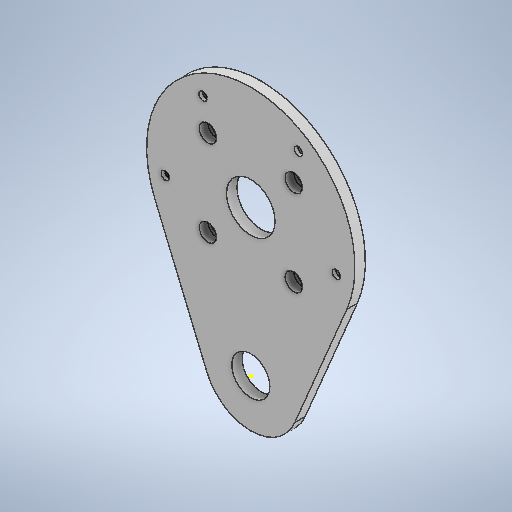
# Autodesk Inventor part: RT_ARM_MC_008_Capstand_Base
Saved by Autodesk Inventor 2025.3 (Build 293356000, 356)
## iProperties
Created: 2026-07-28
Part Number: RT_ARM_MC_008_Capstand_Base
Material: Generic
Document SubType Name: Modeling
Designer: louis
Density: 1 g/cm^3
Appearance: Default
Author: louis
Autodesk Inventor part; units mm, degrees
ref_plane "YZ Plane" through (0, 0, 0) normal (1, 0, 0) x (0, 1, 0)
ref_plane "XZ Plane" through (0, 0, 0) normal (0, 1, 0) x (-1, 0, 0)
ref_plane "XY Plane" through (0, 0, 0) normal (0, 0, 1) x (1, 0, 0)
sketch "Sketch1" plane through (0, 0, 0) normal (0, 0, 1) x (1, 0, 0)
  circle A0 centre (0, 0) radius 11
  circle A1 centre (0, 84) radius 14
  circle A2 centre (0, 0) radius 72 construction
  circle A3 centre (0, 84) radius 12 construction
  line L0 (0, 84) -> (0, 0) construction
  line L1 (-67.6579, 24.6255) -> (0, 0) construction
  line L2 (67.6579, 24.6255) -> (0, 0) construction
  circle A4 centre (0, 84) radius 35 construction
  line L3 (-60, 71.9226) -> (-60, 144)
  line L4 (-60, 144) -> (60, 144)
  line L5 (60, 144) -> (60, 71.9226)
  circle A5 centre (0, 0) radius 27.5
  line L6 (25.3583, -10.6399) -> (60, 71.9226)
  line L7 (-60, 71.9226) -> (-25.3583, -10.6399)
  line L8 (0, 0) -> (135.9462, -63.3927) construction
  line L9 (-24.7487, 59.2513) -> (24.7487, 59.2513) construction
  circle A6 centre (0, 84) radius 60
  point P0 (24.7487, 108.7487)
  point P1 (-24.7487, 108.7487)
  point P2 (55.3272, 60.7857)
  point P3 (-55.3272, 60.7857)
  dimension "d7" = 70
  dimension "d1" = 24
  dimension "d2" = 144
  dimension "d3" = 28
  dimension "d4" = 22
  dimension "d6" = 220
  dimension "d10" = 360
  dimension "d12" = 55
  dimension "d17" = 150
  dimension "d18" = 45
  dimension "d28" = 120
  constraints: 20 end point, 6 centre point, 6 coincident, 6 tangent, 4 point on circle, 2 perpendicular, 2 vertical, 1 horizontal, 10 other
  measures "d1" diameter of A3
  measures "d2" diameter of A2
  measures "d3" diameter of A1
  measures "d4" diameter of A0
  measures "d12" diameter of A5
  measures "d17" distance of L8.start L8.end
  measures "d18" angle of L2 L8
  measures "d28" diameter of A6
sketch "Sketch2" plane through (0, 0, 0) normal (0, 0, 1) x (1, 0, 0)
  point P0 (0, 0)
extrude "Extrusion1" add sketch "Sketch1" against normal blind 6 contours A6 A5 | A6 A5 L7 | A5 A6 | A5 A6 | A5 A6 L6
hole "Hole1" at (-24.7487, 59.2513, 0) at (-24.7487, 108.7487, 0) at (24.7487, 108.7487, 0) at (24.7487, 59.2513, 0) direction (0, 0, -1) diameter 5.8 end through all counterbore diameter 10 counterbore depth 5 clearance for "Socket Head Cap Screw" size "M5" standard "Ansi Metric M Profile"
sketch "Sketch3" plane through (0, 0, -6) normal (0, 0, -1) x (-1, 0, 0)
  circle A0 centre (0, 84) radius 50 construction
  line L0 (0, 84) -> (0, 134) construction
  circle A1 centre (0, 84) radius 14 construction
  line L1 (-49.2404, 75.3176) -> (0, 84) construction
  point P0 (0, 0)
  point P1 (-27.4754, 125.7744)
  point P2 (27.4754, 125.7744)
  point P3 (49.2404, 75.3176)
  dimension "d29" = 100
  dimension "d30" = 100
  dimension "d33" = 200
  constraints: 4 end point, 2 point on circle, 1 centre point, 1 coincident, 1 vertical, 4 other
  measures "d29" diameter of A0
  measures "d30" angle of L0 L1
hole "Hole2" at (0, 84, -6) at (49.2404, 75.3176, -6) at (27.4754, 125.7744, -6) at (-27.4754, 125.7744, -6) at (-49.2404, 75.3176, -6) direction (0, 0, 1) diameter 4.8 end through all counterbore diameter 8 counterbore depth 4 clearance for "Socket Head Cap Screw" size "M4" standard "Ansi Metric M Profile"
equation "\"d2\" = 6 * d1"
body "Solid1"
